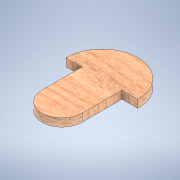
# Autodesk Inventor part: Parte D
Saved by Autodesk Inventor 2022 (Build 260153000, 153)
## iProperties
Created: 2023-02-12
Part Number: Parte D
Material: Madera (abedul)
Document SubType Name: Modeling
Designer: USUARIO
Density: 0.55 g/cm^3
Appearance: Abedul - Natural pulido
Author: USUARIO
Autodesk Inventor part; units mm, degrees
ref_plane "YZ Plane" through (0, 0, 0) normal (1, 0, 0) x (0, 1, 0)
ref_plane "XZ Plane" through (0, 0, 0) normal (0, 1, 0) x (-1, 0, 0)
ref_plane "XY Plane" through (0, 0, 0) normal (0, 0, 1) x (1, 0, 0)
sketch "Boceto1" plane through (0, 0, 0) normal (0, 1, 0) x (-1, 0, 0)
  arc A0 (-45, 0) -> (45, 0) centre (0, 0) ccw
  line L0 (45, 0) -> (-45, 0)
  line L1 (25, -50) -> (-25, -50)
  line L2 (-25, -50) -> (-25, 50)
  line L3 (-25, 50) -> (25, 50)
  line L4 (25, 50) -> (25, -50)
  line L5 (25, -50) -> (-25, 50) construction
  line L6 (-25, -50) -> (25, 50) construction
  circle A1 centre (0, 50) radius 25
  point P0 (25, 0)
  point P1 (25, 50)
  point P2 (-25, 0)
  dimension "d0" = 90
  dimension "d1" = 50
  dimension "d2" = 100
  constraints: 14 end point, 3 midpoint, 2 horizontal, 2 parallel, 2 point on circle, 1 centre point, 1 coincident, 1 perpendicular, 3 other
  measures "d0" diameter of A0
  measures "d1" distance of L2.end L3.end
  measures "d2" distance of L1.end L2.end
extrude "Extrusión1" add sketch "Boceto1" along normal blind 10 contours L0 L2 A0 | L2 L0 L4 A0 | L2 A1 L4 L0 | L4 L0 A0 | A1 L3 | L3 A1
equation "\"d0\" = diametro_c"
equation "\"d1\" = ancho_p"
equation "\"d2\" = largo_p"
equation "\"d3\" = grueso"
equation "\"diametro_c\" = 90"
equation "\"grueso\" = 10"
equation "\"ancho_p\" = 50"
equation "\"largo_p\" = 100"
